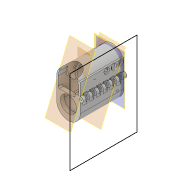
# Autodesk Inventor part: cellSTORM_objective_tube_folded_mirror_v0
Saved by Autodesk Inventor 2019 (Build 230136000, 136)
## iProperties
Created: 2019-11-14
Part Number: cellSTORM_objective_tube_folded_mirror_v0
Material: Generic
Document SubType Name: Modeling
Designer: diederichbenedict
Density: 1 g/cm^3
Appearance: Default
Author: diederichbenedict
Autodesk Inventor part; units mm, degrees
ref_plane "YZ Plane" through (0, 0, 0) normal (1, 0, 0) x (0, 1, 0)
ref_plane "XZ Plane" through (0, 0, 0) normal (0, 1, 0) x (-1, 0, 0)
ref_plane "XY Plane" through (0, 0, 0) normal (0, 0, 1) x (1, 0, 0)
ref_plane "Work Plane1" through (18.16385, -15, -12.5) normal (0, 0, 1) x (1, 0, 0)
sketch "Sketch1" plane through (18.16385, -15, -12.5) normal (0, 0, 1) x (1, 0, 0)
  circle A0 centre (0, 14.999991) radius 17.5
  circle A1 centre (0, 14.999991) radius 10.375
  line L0 (-2.148982, 25.149991) -> (2.148982, 25.149991)
  dimension "d125" = 20.75
  dimension "d126" = 35
  dimension "d128" = 10.15
  constraints: 2 centre point, 2 end point, 2 point on circle, 1 coincident, 1 horizontal
  measures "d125" diameter of A1
  measures "d126" diameter of A0
  measures "d128" distance from line of L0 A0.centre
extrude "Extrusion1" add sketch "Sketch1" along normal blind 5 contours A0 | L0 A1 picked at (0.240323, 25.216631)
pattern_circular "Circular Pattern1" count 3 over 360 about axis through (18.16385, -0.000009, -12.5) along (0, 0, 1) of "Extrusion1"
sketch "Sketch2" plane through (18.16385, -0.000009, -12.5) normal (0, 0, -1) x (-1, 0, 0)
  circle A0 centre (0, 0) radius 17.5 projected
  line L0 (17.5, 0) -> (17.5, -32)
  line L1 (-17.5, 0) -> (-17.5, -32)
  arc A1 (-17.5, -32) -> (17.5, -32) centre (0, -32) ccw
  point P0 (18.16385, 0.000009)
  dimension "d9" = 32
  constraints: 4 end point, 4 point on circle, 2 tangent, 2 vertical, 1 centre point
  measures "d9" distance of L0.start L0.end
extrude "Extrusion2" add sketch "Sketch2" against normal up to surface (5 mm away) contours L0 A1 L1 A0
sketch "Sketch3" plane through (18.16385, -15, -7.5) normal (0, 0, 1) x (1, 0, 0)
  arc A0 (17.5, 14.999991) -> (-17.5, 14.999991) centre (0, 14.999991) ccw
  line L0 (-17.5, 14.999991) -> (-17.5, -17.000009)
  arc A1 (-17.5, -17.000009) -> (17.5, -17.000009) centre (0, -17.000009) ccw
  line L1 (17.5, -17.000009) -> (17.5, 14.999991)
  line L2 (-15.5, -17.000009) -> (-15.5, 14.999991)
  arc A2 (15.5, 14.999991) -> (-15.5, 14.999991) centre (0, 14.999991) ccw
  line L3 (15.5, 14.999991) -> (15.5, -17.000009)
  arc A3 (-15.5, -17.000009) -> (15.5, -17.000009) centre (0, -17.000009) ccw
  point P0 (-18.16385, 15)
  dimension "d12" = 2
  constraints: 4 end point, 4 point on circle, 2 centre point, 3 other
  measures "d12" distance between parallel lines of L0 L2
extrude "Extrusion3" add sketch "Sketch3" along normal blind 60
sketch "Sketch4" plane through (18.16385, -15, -7.5) normal (0, 0, 1) x (1, 0, 0)
  arc A0 (15.5, 14.999991) -> (-15.5, 14.999991) centre (0, 14.999991) ccw construction
  line L0 (-15.5, 14.999991) -> (-15.5, -17.000009) construction
  arc A1 (-15.5, -17.000009) -> (15.5, -17.000009) centre (0, -17.000009) ccw
  line L1 (15.5, -17.000009) -> (15.5, 14.999991) construction
  line L2 (-15.5, 14.999991) -> (-15.5, -17.000009) construction
  line L3 (15.5, -17.000009) -> (15.5, 14.999991) construction
  line L4 (-15.5, -1.000009) -> (15.5, -1.000009)
  line L5 (-15.5, -17.000009) -> (-15.5, -1.000009) construction
  line L6 (-15.5, -17.000009) -> (-15.5, -1.000009)
  line L7 (15.5, -1.000009) -> (15.5, -17.000009)
  point P0 (-18.16385, 15)
  point P1 (15.5, -27.879426)
  point P2 (15.5, -7.648413)
  constraints: 8 end point, 2 collinear, 2 midpoint, 2 point on line, 1 vertical
extrude "Extrusion4" add sketch "Sketch4" along normal blind 10
ref_plane "Work Plane2" through (33.66385, -16.000009, 2.5) normal (0, 0.3826834, 0.9238795) x (-1, 0, 0)
sketch "Sketch5" plane through (33.66385, -16.000009, 2.5) normal (0, 0.3826834, 0.9238795) x (-1, 0, 0)
  circle A0 centre (15.5, 10.475034) radius 12.45
  circle A1 centre (15.5, 10.475034) radius 12.7
  circle A2 centre (15.5, 10.475034) radius 13.7
  point P0 (33.66385, -15.73879)
  dimension "d18" = 1
  constraints: 1 centre point
  measures "d18" radial gap between concentric circles of A1 A2
extrude "Extrusion5" cut sketch "Sketch5" along normal blind 24 and the other way blind 13 contours A0 | A1 | A2
sketch "Sketch6" plane through (35.66385, -32.000009, -12.5) normal (1, 0, 0) x (0, 0, -1)
  line L0 (-80.533836, -65.200836) -> (19.238431, -65.200836)
  line L1 (19.238431, -65.200836) -> (19.238431, 59.59269)
  line L2 (19.238431, 59.59269) -> (-80.533836, 59.59269)
  line L3 (-80.533836, 59.59269) -> (-80.533836, -65.200836)
  point P0 (-12.5, 32.000009)
  constraints: 8 end point, 2 parallel, 1 horizontal, 1 perpendicular
ref_plane "Work Plane3" through (18.16385, -15, 20.5) normal (0, 0, 1) x (1, 0, 0)
sketch "Sketch7" plane through (18.16385, -15, 20.5) normal (0, 0, 1) x (1, 0, 0)
  arc A0 (15.5, 14.999991) -> (-15.5, 14.999991) centre (0, 14.999991) ccw
  line L0 (-15.5, -17.000009) -> (-15.5, 14.999991)
  line L1 (15.5, 14.999991) -> (15.5, -17.000009)
  line L2 (-15.5, 14.999991) -> (15.5, 14.999991)
  line L3 (15.5, 14.999991) -> (15.5, 5.999991)
  line L4 (15.5, 5.999991) -> (-15.5, 5.999991)
  line L5 (-15.5, 5.999991) -> (-15.5, 14.999991)
  arc A1 (15.5, 14.999991) -> (-15.5, 14.999991) centre (0, 14.999991) ccw
  point P0 (-18.16385, 15)
  point P1 (0, 30.5)
  dimension "d26" = 9
  constraints: 8 end point, 2 parallel, 2 point on circle, 2 tangent, 1 centre point, 1 horizontal, 1 perpendicular, 1 point on line
  measures "d26" distance of L2.end L3.end
extrude "Extrusion7" add sketch "Sketch7" along normal blind 20
ref_plane "Work Plane4" through (33.66385, 2.560137, 47.308157) normal (0, 0.3826834, 0.9238795) x (-1, 0, 0)
sketch "Sketch8" plane through (33.66385, 2.560137, 47.308157) normal (0, 0.3826834, 0.9238795) x (-1, 0, 0)
  circle A0 centre (15.5, -4.832303) radius 12.7
  circle A1 centre (15.5, -4.832303) radius 13.2
  point P0 (33.66385, -15.73879)
  dimension "d36" = 0.5
  constraints: 1 centre point
  measures "d36" radial gap between concentric circles of A0 A1
extrude "Extrusion8" cut sketch "Sketch8" along normal blind 28.5 and the other way blind 18.5 contours A0 | A1
chamfer "Chamfer1" distance 5 angle 45 2 edges at (9.0312, -9, 40.5) (27.2964, -9, 40.5)
sketch "Sketch10" plane through (18.16385, -15, 52.5) normal (0, 0, 1) x (1, 0, 0)
  circle A0 centre (0, 15) radius 10 projected
  circle A1 centre (0, 15) radius 10
  point P0 (-18.16385, 15)
  constraints: 1 centre point, 1 coincident, 1 concentric
ref_plane "Work Plane5" through (-23.920278, -14.5, 0) normal (0, 0, 1) x (1, 0, 0)
extrude "Extrusion10" cut sketch "Sketch10" against normal up to surface (52.5 mm away)
sketch "Sketch11" plane through (0.66385, -32.000009, -12.5) normal (-1, 0, 0) x (0, 0, 1)
  line L0 (6, 46.5) -> (6, 17.5) construction
  line L1 (6, 17.5) -> (12.5, 17.5) construction
  line L2 (12.5, 46.5) -> (12.5, 17.5) construction
  line L3 (6, 46.5) -> (12.5, 46.5) construction
  line L4 (12.5, 46.5) -> (6, 17.5) construction
  line L5 (12.5, 17.5) -> (6, 46.5) construction
  line L6 (0, 26.26449) -> (0, 44.284483) construction
  line L7 (0, 26.26449) -> (5, 26.26449) construction
  line L8 (5, 44.284483) -> (5, 26.26449) construction
  line L9 (0, 44.284483) -> (5, 44.284483) construction
  line L10 (0, 19.5) -> (0, 27.859284) construction
  line L11 (0, 49.5) -> (0, 32) construction
  line L12 (14.75, 16.75) -> (3.75, 16.75) construction
  line L13 (3.75, 16.75) -> (3.75, 47.25) construction
  line L14 (3.75, 47.25) -> (14.75, 47.25) construction
  line L15 (14.75, 47.25) -> (14.75, 16.75) construction
  line L16 (14.75, 16.75) -> (3.75, 47.25) construction
  line L17 (3.75, 16.75) -> (14.75, 47.25) construction
  line L18 (16, 47.25) -> (5, 47.25)
  line L19 (5, 47.25) -> (5, 16.75)
  line L20 (5, 16.75) -> (16, 16.75)
  line L21 (16, 16.75) -> (16, 47.25)
  line L22 (5, 16) -> (5, 32) construction
  point P0 (9.25, 32)
  point P1 (0, 19.675118)
  point P2 (9.25, 32)
  dimension "d95" = 11
  dimension "d96" = 30.5
  dimension "d97" = 11
  dimension "d98" = 30.5
  dimension "d99" = 0
  constraints: 24 end point, 4 parallel, 3 midpoint, 2 horizontal, 2 perpendicular, 1 coincident
  measures "d95" distance of L13.end L14.end
  measures "d96" distance of L12.end L13.end
  measures "d97" distance of L20.end L19.end
  measures "d98" distance of L19.end L18.end
  measures "d99" distance between parallel lines of L22 L19
extrude "Extrusion11" cut sketch "Sketch11" against normal blind 20
sketch "Sketch13" plane through (18.16385, -15, 52.5) normal (0, 0, 1) x (1, 0, 0)
  circle A0 centre (0, -13.284271) radius 11.5 construction
  circle A1 centre (0, -13.284271) radius 12
  arc A2 (-15.5, -17.000009) -> (15.5, -17.000009) centre (0, -17.000009) ccw
  arc A3 (-17.5, -17.000009) -> (17.5, -17.000009) centre (0, -17.000009) ccw
  ellipse E0 centre (0, 24.941116) end of major axis (0, 39.228693) minor radius 13.2 (-13.111789, 26.590115) -> (-13.109402, 23.270031) ccw
  arc A4 (-13.111789, 26.590115) -> (-17.5, 14.999991) centre (0, 14.999991) ccw
  line L0 (-17.5, 14.999991) -> (-17.5, -17.000009)
  arc A5 (-17.5, -17.000009) -> (17.5, -17.000009) centre (0, -17.000009) ccw
  line L1 (17.5, -17.000009) -> (17.5, 14.999991)
  arc A6 (17.5, 14.999991) -> (13.111789, 26.590115) centre (0, 14.999991) ccw
  ellipse E1 centre (0, 24.941116) end of major axis (0, 39.228693) minor radius 13.2 (13.109402, 23.270031) -> (13.111789, 26.590115) ccw
  arc A7 (15.5, 14.999991) -> (13.109402, 23.270031) centre (0, 14.999991) ccw
  line L2 (15.5, 14.999991) -> (15.5, -17.000009)
  arc A8 (-15.5, -17.000009) -> (15.5, -17.000009) centre (0, -17.000009) ccw
  line L3 (-15.5, -17.000009) -> (-15.5, 14.999991)
  arc A9 (-13.109402, 23.270031) -> (-15.5, 14.999991) centre (0, 14.999991) ccw
  line L4 (15.5, -1.000009) -> (15.5, -17.000009)
  line L5 (-15.5, -17.000009) -> (-15.5, -1.000009)
  line L6 (-15.5, -7.28492) -> (-10.392679, -7.28492)
  line L7 (10.392679, -7.28492) -> (15.5, -7.28492)
  point P0 (-18.16385, 15)
  point P1 (15.5, -9.000009)
  point P2 (11.273156, -9.171371)
  point P3 (-15.5, -9.000009)
  point P4 (-11.273156, -9.171371)
  dimension "d48" = 0.5
  constraints: 4 end point, 4 point on circle, 4 point on line, 2 midpoint, 1 centre point, 1 perpendicular, 2 other
  measures "d48" radial gap between concentric circles of A0 A1
extrude "Extrusion13" add sketch "Sketch13" against normal blind 3 contours A1 L7 L2 A2 L3 L6 | L2 A7 E1 A6 L1 A3 L0 A4 E0 A9 L3 A2
chamfer "Chamfer2" distance 5 angle 45 6 edges at (33.6638, -27.1425, 49.5) (18.1638, -47.5, 49.5) (2.6638, -27.1425, 49.5) (33.6638, -4.5, 20.5) (18.1638, 15.5, 20.5) (2.6638, -4.5, 20.5)
sketch "Sketch14" plane through (18.16385, -15, 52.5) normal (0, 0, 1) x (1, 0, 0)
  line L0 (17.950115, 6.5) -> (22.950115, 6.5) construction
  line L1 (22.950115, -3.5) -> (17.950115, -3.5) construction
  circle A0 centre (17.950115, 1.5) radius 1.55 construction
  arc A1 (17.950115, -2.5) -> (17.950115, 5.5) centre (17.950115, 1.5) ccw construction
  line L2 (17.950115, 5.5) -> (12.546472, 5.5) construction
  line L3 (17.950115, 5.5) -> (9.950115, 5.5) construction
  line L4 (9.950115, 5.5) -> (9.950115, -2.5) construction
  line L5 (9.950115, -2.5) -> (17.950115, -2.5) construction
  line L6 (17.950115, -2.5) -> (17.950115, -0.05) construction
  line L7 (17.950115, -2.5) -> (17.950115, -0.05) construction
  line L8 (17.950115, 5.5) -> (9.950115, 5.5) construction
  line L9 (17.950115, 5.5) -> (9.950115, 5.5)
  line L10 (9.950115, 5.5) -> (9.950115, -2.5)
  line L11 (9.950115, -2.5) -> (17.950115, -2.5)
  arc A2 (17.950115, -2.5) -> (17.950115, 5.5) centre (17.950115, 1.5) ccw
  line L12 (10.392679, -7.28492) -> (9.950115, -2.5)
  line L13 (10.392679, -7.28492) -> (15.108653, -7.28492)
  line L14 (15.108653, -7.28492) -> (15.5, -2.5)
  line L15 (15.5, -1.000009) -> (15.5, -17.000009)
  point P0 (-18.16385, 15)
  dimension "d54" = 4
  dimension "d55" = 8
  constraints: 26 end point, 4 collinear, 4 point on circle, 3 horizontal, 2 centre point, 2 parallel, 2 perpendicular, 2 point on line, 2 tangent, 1 coincident, 1 vertical alignment, 1 other
  measures "d54" radius of A1
  measures "d55" distance of L5.end L4.end
extrude "Extrusion14" add sketch "Sketch14" against normal up to surface (65 mm away)
sketch "Sketch15" plane through (18.16385, -15, 52.5) normal (0, 0, 1) x (1, 0, 0)
  circle A0 centre (17.950115, 1.5) radius 1.55
  point P0 (-18.16385, 15)
extrude "Extrusion15" cut sketch "Sketch15" against normal through all
ref_plane "Work Plane6" through (18.16385, -15, -7.5) normal (0, 0, -1) x (-1, 0, 0)
sketch "Sketch17" plane through (18.16385, -30.652564, -5.501812) normal (0, 0.3826834, 0.9238795) x (1, 0, 0)
  circle A0 centre (0, 0) radius 13.7 projected
  point P0 (-18.16385, 26.213824)
extrude "Extrusion17" cut sketch "Sketch17" along normal blind 30
sketch "Sketch16" plane through (18.16385, -15, -7.5) normal (0, 0, -1) x (-1, 0, 0)
  line L0 (-17.950115, -3.5) -> (-22.950115, -3.5) construction
  arc A0 (-17.950115, -3.5) -> (-17.950115, 6.5) centre (-17.950115, 1.5) ccw construction
  line L1 (-22.950115, 6.5) -> (-17.950115, 6.5) construction
  line L2 (-22.950115, -4) -> (-17.950115, -4)
  arc A1 (-17.950115, -4) -> (-17.950115, 7) centre (-17.950115, 1.5) ccw
  line L3 (-17.950115, 7) -> (-22.950115, 7)
  line L4 (-22.950115, -4) -> (-22.950115, 7)
  line L5 (-22.950115, -4) -> (-22.950115, -17.034383)
  line L6 (-22.950115, -17.034383) -> (-13.940231, -2.264416)
  point P0 (18.16385, 15)
  dimension "d61" = 0.5
  constraints: 10 end point, 3 point on circle, 2 vertical, 1 centre point, 2 other
  measures "d61" distance between parallel lines of L0 L2
extrude "Extrusion16" cut sketch "Sketch16" against normal blind 6
pattern_linear "Rectangular Pattern1" count 6 spacing 10 along (0, 0, 1) of "Extrusion16"
sketch "Sketch18" plane through (0.66385, -32.000009, -12.5) normal (-1, 0, 0) x (0, 0, 1)
  line L0 (41.452228, 45.9337) -> (51.172387, 22.46716)
  line L1 (51.307686, 22.7938) -> (41.778868, 45.798401)
  line L2 (84.015729, 117.715729) -> (84.015729, -22.284271)
  line L3 (46.091049, 20.362401) -> (36.37089, 43.828941)
  circle A0 centre (43.343205, 34.296101) radius 1.4
  line L4 (17.480137, -7.786571) -> (7.95132, 15.218029)
  line L5 (15, 16) -> (15, -10.166868)
  line L6 (6.572758, 16) -> (15, 16)
  line L7 (1.755425, 14.004595) -> (12.240951, -11.309704)
  circle A1 centre (9.867033, 2.53576) radius 1.4
  point P0 (12.5, 32.000009)
  point P1 (15, 9.715089)
  dimension "d72" = 2.8
  dimension "d75" = 2.8
  constraints: 2 centre point
  measures "d72" diameter of A0
  measures "d75" diameter of A1
extrude "Extrusion18" cut sketch "Sketch18" against normal through all
sketch "Sketch19" plane through (18.16385, -15, 52.5) normal (0, 0, 1) x (1, 0, 0)
  arc A0 (15.5, 14.999991) -> (13.109402, 23.270031) centre (0, 14.999991) ccw
  arc A1 (17.5, 14.999991) -> (13.111789, 26.590115) centre (0, 14.999991) ccw
  line L0 (17.5, 14.999991) -> (17.5, 23.457014)
  line L1 (17.5, 23.457014) -> (15.32086, 23.457014)
  point P0 (-18.16385, 15)
  constraints: 4 end point, 1 perpendicular, 1 point on circle, 1 vertical
extrude "Extrusion19" add sketch "Sketch19" against normal up to surface (65 mm away)
sketch "Sketch20" plane through (35.66385, -9.5, -7.5) normal (1, 0, 0) x (0, 0, -1)
  circle A0 centre (-10.2, 13.2) radius 4.5
  circle A1 centre (-10.2, 13.2) radius 4.05
  circle A2 centre (-20.750802, 13.2) radius 4.05
  circle A3 centre (-0.0056, 13.2) radius 4.05
  point P0 (-7.5, 9.5)
  dimension "d78" = 8.1
  dimension "d84" = 8.1
  dimension "d85" = 8.1
  constraints: 3 centre point, 1 coincident
  measures "d78" diameter of A1
  measures "d84" diameter of A2
  measures "d85" diameter of A3
extrude "Extrusion20" cut sketch "Sketch20" against normal blind 3 contours A1 | A2 | A3
ref_plane "Work Plane7" through (0.66385, -15.5, 1) normal (0, 0, -1) x (-1, 0, 0)
sketch "Sketch27" plane through (18.16385, -15, -7.5) normal (0, 0, 1) x (1, 0, 0)
  circle A0 centre (17.950115, 1.5) radius 1.55
  line L0 (17.5, -2.5) -> (17.5, -17.000009)
  arc A1 (-17.5, -17.000009) -> (17.5, -17.000009) centre (0, -17.000009) ccw
  line L1 (-17.5, -17.000009) -> (-17.5, 14.999991)
  arc A2 (15.32086, 23.457014) -> (-17.5, 14.999991) centre (0, 14.999991) ccw
  line L2 (15.32086, 23.457014) -> (17.5, 23.457014)
  line L3 (17.5, 23.457014) -> (17.5, 5.5)
  line L4 (17.950115, 5.5) -> (17.5, 5.5)
  arc A3 (17.950115, -2.5) -> (17.950115, 5.5) centre (17.950115, 1.5) ccw
  line L5 (17.5, -2.5) -> (17.950115, -2.5)
  circle A4 centre (0, 14.999991) radius 15.25
  point P0 (-18.16385, 15)
  dimension "d100" = 30.5
  constraints: 1 centre point, 1 coincident
  measures "d100" diameter of A4
extrude "Extrusion25" cut sketch "Sketch27" along normal up to surface (11 mm away) contours A4
sketch "Sketch28" plane through (18.16385, -15, -7.5) normal (0, 0, 1) x (1, 0, 0)
  circle A0 centre (17.950115, 1.5) radius 1.55 construction
  line L0 (11.929488, 5.5) -> (14.175198, 5.5) construction
  arc A1 (14.175198, 5.5) -> (13.940231, -2.264416) centre (17.950115, 1.5) ccw construction
  line L1 (17.5, -8.09997) -> (13.940231, -2.264416) construction
  line L2 (17.5, -2.5) -> (17.5, -8.09997) construction
  line L3 (17.950115, -2.5) -> (17.5, -2.5) construction
  arc A2 (17.950115, -2.5) -> (17.950115, 5.5) centre (17.950115, 1.5) ccw construction
  line L4 (17.5, 5.5) -> (17.950115, 5.5) construction
  line L5 (17.5, 6.981551) -> (17.5, 5.5) construction
  arc A3 (17.5, 6.981551) -> (15.5, 6.424118) centre (17.950115, 1.5) ccw construction
  line L6 (15.5, 6.424118) -> (15.5, 14.650004) construction
  line L7 (15.5, 14.650004) -> (14.5, 14.650004) construction
  line L8 (14.5, 14.650004) -> (14.5, 20.477216) construction
  arc A4 (14.5, 20.477216) -> (-2.772634, 30.249991) centre (0, 14.999991) ccw construction
  line L9 (-8.584142, 30.249991) -> (-2.772634, 30.249991) construction
  arc A5 (-8.584142, 30.249991) -> (-17.5, 14.999991) centre (0, 14.999991) ccw construction
  line L10 (-17.5, -0.250009) -> (-17.5, 14.999991) construction
  line L11 (-17.5, -0.250009) -> (-15.5, -0.250009) construction
  line L12 (-15.5, -0.250009) -> (-15.5, -1.000009) construction
  line L13 (-15.5, -1.000009) -> (9.950115, -1.000009) construction
  line L14 (9.950115, -1.000009) -> (9.950115, 3.443274) construction
  circle A6 centre (0, 14.999991) radius 15.25 construction
  arc A7 (-8.584142, 30.249991) -> (-17.5, 14.999991) centre (0, 14.999991) ccw construction
  line L15 (-8.584142, 30.249991) -> (0, 30.249991) construction
  line L16 (-17.5, -0.250009) -> (0, -0.250009) construction
  line L17 (9.950115, -1.000009) -> (9.950115, 3.443274) construction
  line L18 (9.950115, 3.4437) -> (9.950115, -1.000009) construction
  line L19 (9.950115, -1.000009) -> (-15.5, -1.000009) construction
  line L20 (-15.5, -1.000009) -> (-15.5, -0.250009) construction
  line L21 (-15.5, -0.250009) -> (-15.483201, -0.250009) construction
  arc A8 (14.5, 20.477216) -> (-2.772634, 30.249991) centre (0, 14.999991) ccw construction
  arc A9 (15.496048, 14.650004) -> (-2.772634, 30.249991) centre (0, 14.999991) ccw construction
  line L22 (15.5, 14.650004) -> (15.5, 14.999991) construction
  line L23 (15.5, 14.650004) -> (15.5, 5.5) construction
  line L24 (15.5, 14.650004) -> (24.650004, 14.650004) construction
  arc A10 (9.950115, 3.443274) -> (11.929488, 5.5) centre (0, 14.999991) ccw construction
  line L25 (15.5, 5.5) -> (11.929488, 5.5) construction
  arc A11 (0, -0.250009) -> (9.950115, 3.4437) centre (0, 14.998656) ccw
  line L26 (9.950115, 3.4437) -> (9.950115, -1.000009)
  line L27 (9.950115, -1.000009) -> (-17.5, -1.000009)
  line L28 (-17.5, -1.000009) -> (-17.5, -0.250009)
  line L29 (-17.5, -0.250009) -> (0, -0.250009)
  arc A12 (11.929488, 5.5) -> (0, 30.249991) centre (0, 14.999991) ccw
  arc A13 (15.496048, 14.650004) -> (0, 30.499991) centre (0, 14.999991) ccw
  line L30 (15.496048, 14.650004) -> (15.5, 5.5)
  line L31 (11.929488, 5.5) -> (15.5, 5.5)
  line L32 (0, 30.499991) -> (0, 30.249991)
  arc A14 (9.950115, 3.443274) -> (11.929488, 5.5) centre (0, 14.999991) ccw
  point P0 (-18.16385, 15)
  point P1 (9.950115, 5.5)
  dimension "d103" = 30.5
  dimension "d104" = 90
  constraints: 32 end point, 11 point on circle, 7 perpendicular, 5 centre point, 3 point on line, 3 tangent, 1 coincident, 1 collinear, 1 concentric, 1 horizontal
  measures "d103" diameter of A6
  measures "d104" angle of L23 L24
extrude "Extrusion26" add sketch "Sketch28" along normal blind 11
ref_plane "Work Plane8" through (0.66385, -15.000009, 5) normal (0, 0, 1) x (1, 0, 0)
sketch "Sketch31" plane through (18.16385, -30.652564, -5.501812) normal (0, 0.3826834, 0.9238795) x (1, 0, 0)
  circle A0 centre (0, 0) radius 13.7 projected
  point P0 (-18.16385, 26.213824)
extrude "Extrusion29" cut sketch "Sketch31" along normal blind 30
sketch "Sketch32" plane through (18.16385, -15, 52.5) normal (0, 0, 1) x (1, 0, 0)
  arc A0 (-10.392679, -7.28492) -> (10.392679, -7.28492) centre (0, -13.284271) ccw
  circle A1 centre (0, -13.284271) radius 12
  line L0 (9.950115, 5.5) -> (9.950115, -2.5)
  line L1 (9.950115, -2.5) -> (10.392679, -7.28492)
  line L2 (-10.392679, -7.28492) -> (-15.5, -7.28492)
  line L3 (-15.5, -7.28492) -> (-15.5, 14.999991)
  line L4 (9.950115, 0.034991) -> (-15.5, 0.034991)
  arc A2 (-14.985199, -20.96155) -> (14.985199, -20.96155) centre (0, -17.000009) ccw
  spline S0 degree 2 poles (15.5, -17.000009) (15.5, -19.014229) (14.985199, -20.96155) knots 0 0 0 1 1 1 weights 1 0.94892244 0.91565968
  arc A3 (-15.5, -17.000009) -> (15.5, -17.000009) centre (0, -17.000009) ccw
  line L5 (15.5, -7.474796) -> (15.5, -17.000009)
  line L6 (15.5, -4.821356) -> (15.5, -2.5)
  line L7 (15.5, -2.5) -> (15.5, -4.821356)
  line L8 (15.5, -4.821356) -> (15.5, -2.5)
  line L9 (15.5, -2.5) -> (15.5, -4.821356)
  line L10 (15.5, -4.821356) -> (15.5, -2.5)
  line L11 (15.5, -2.5) -> (15.5, -4.821356)
  line L12 (15.5, -4.821356) -> (15.5, -2.5)
  line L13 (15.5, -2.5) -> (15.5, -4.821356)
  line L14 (15.5, -4.821356) -> (15.5, -17.000009)
  line L15 (15.5, -7.474796) -> (15.5, -17.000009)
  line L16 (15.5, -7.28492) -> (15.5, -7.474796)
  line L17 (15.5, -2.5) -> (15.5, -7.28492)
  line L18 (15.5, -2.5) -> (15.5, -4.821356)
  line L19 (-15.5, 5.999991) -> (-15.5, 14.999991)
  line L20 (-15.5, 10.999991) -> (-15.5, 5.999991)
  line L21 (-15.5, 10.999991) -> (-15.5, 14.999991)
  line L22 (-15.5, -7.28492) -> (-15.5, 14.999991)
  line L23 (-15.5, -7.474796) -> (-15.5, -7.28492)
  line L24 (-15.5, -17.000009) -> (-15.5, -7.474796)
  line L25 (-15.5, -17.000009) -> (-15.5, -1.000009)
  line L26 (-15.5, -1.000009) -> (-15.5, -0.250009)
  line L27 (-15.5, -0.250009) -> (-15.5, 14.999991)
  line L28 (9.950115, 5.5) -> (15.5, -2.240097)
  line L29 (15.5, -2.240097) -> (15.5, -2.5)
  arc A4 (-15.5, -17.000009) -> (15.5, -17.000009) centre (0, -17.000009) ccw
  line L30 (15.5, -2.5) -> (15.5, -17.000009)
  line L31 (9.950115, 0.034991) -> (13.868693, 0.034991)
  line L32 (-15.5, 0.034991) -> (-15.5, -17.000009)
  arc A5 (-15.5, -17.000009) -> (15.5, -17.000009) centre (0, -17.000009) ccw
  point P0 (-18.16385, 15)
  constraints: 12 end point, 3 point on line, 3 tangent, 2 centre point, 2 coincident, 2 perpendicular, 2 point on circle, 2 vertical, 1 collinear, 1 concentric, 1 horizontal, 3 other
extrude "Extrusion30" add sketch "Sketch32" against normal blind 6 contours L2 L3 L4 L0 L1 A1 | A0 L1 L0 L31 L28 L29 L6 L14 L5 S0 A2 A3 L24 L23 L2 | L0 L28 L31
fillet "Fillet1" radius 2 2 edges at (28.114, -14.965, 49.5) (2.6638, -14.965, 49.5)
body "Solid1"
